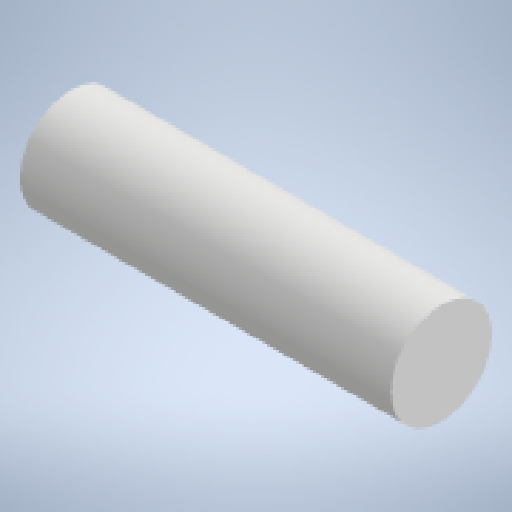
# Autodesk Inventor part: AA
Saved by Autodesk Inventor 2025 (Build 290162010, 162A)
## iProperties
Created: 2025-02-03
Part Number: AA
Material: Generisch
Document SubType Name: Modeling
Designer: Admin
Density: 1 g/cm^3
Appearance: Vorgabe
Author: Admin
Autodesk Inventor part; units mm, degrees
ref_plane "YZ Plane" through (0, 0, 0) normal (1, 0, 0) x (0, 1, 0)
ref_plane "XZ Plane" through (0, 0, 0) normal (0, 1, 0) x (-1, 0, 0)
ref_plane "XY Plane" through (0, 0, 0) normal (0, 0, 1) x (1, 0, 0)
sketch "Skizze1" plane through (0, 0, 0) normal (1, 0, 0) x (0, 1, 0)
  circle A0 centre (0, 0) radius 7.5
  circle A1 centre (15, 0) radius 7.5
  circle A2 centre (30, 0) radius 7.5
  line L0 (-7.5, 0) -> (37.5, 0)
  line L1 (37.5, 0) -> (37.5, -7.5)
  line L2 (37.5, -7.5) -> (-7.5, -7.5)
  line L3 (-7.5, -7.5) -> (-7.5, 0)
  point P0 (22.5, 0)
  point P1 (7.5, 0)
  point P2 (0, -7.5)
  dimension "d0" = 15
  dimension "d3" = 15
  dimension "d4" = 15
  dimension "d5" = 15
  dimension "d6" = 15
  constraints: 8 end point, 2 centre point, 2 parallel, 1 coincident, 1 horizontal, 1 perpendicular, 3 other
  measures "d3" diameter of A1
  measures "d4" diameter of A2
  measures "d5" distance of A1.centre point (0, 0)
  measures "d6" distance of A2.centre A1.centre
extrude "Extrusion1" add sketch "Skizze1" along normal blind 55
